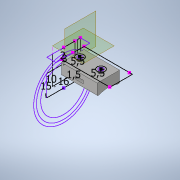
# Autodesk Inventor part: OBS-Displaymountadapter_schmal
Saved by Autodesk Inventor 2021.1 (Build 251245010, 245A)
## iProperties
Created: 2020-11-13
Part Number: OBS-Displaymountadapter_schmal
Material: Generic
Document SubType Name: Modeling
Designer: Administrator
Density: 1 g/cm^3
Appearance: Default
Title: OBS-D-003 v13
Author: Administrator
Autodesk Inventor part; units mm, degrees
ref_plane "YZ Plane" through (0, 0, 0) normal (1, 0, 0) x (0, 1, 0)
ref_plane "XZ Plane" through (0, 0, 0) normal (0, 1, 0) x (-1, 0, 0)
ref_plane "XY Plane" through (0, 0, 0) normal (0, 0, 1) x (1, 0, 0)
ref_plane "Arbeitsebene1" through (-0.5, 0, -8) normal (0, -1, 0) x (1, 0, 0)
sketch "Skizze1" plane through (-0.5, 0, -8) normal (0, -1, 0) x (1, 0, 0)
  line L0 (-6.1, 20) -> (0.5, 20)
  line L1 (0.5, 20) -> (0.5, -4)
  line L2 (0.5, -4) -> (-6.1, -4)
  line L3 (-6.1, -4) -> (-6.1, 20)
  line L4 (0.5, 0) -> (32.9, 0) projected
  line L5 (0.5, 16) -> (34.9, 16) projected
  line L6 (0.5, 0) -> (34.9, 0)
  line L7 (34.9, 0) -> (34.9, 16)
  line L8 (34.9, 16) -> (0.5, 16)
  line L9 (0.5, 16) -> (0.5, 0)
  circle A0 centre (5.5, 8) radius 1.6 projected
  circle A1 centre (5.5, 8) radius 1.6
  circle A2 centre (20.5, 8) radius 1.6 projected
  circle A3 centre (20.5, 8) radius 1.6
  circle A4 centre (5.5, 8) radius 2.75
  circle A5 centre (20.5, 8) radius 2.75
  point P0 (0.5, 8)
  dimension "d0" = 5.5
  dimension "d1" = 5.5
  constraints: 16 end point, 4 centre point, 4 coincident, 4 parallel, 2 horizontal, 2 perpendicular
  measures "d0" diameter of A4
  measures "d1" diameter of A5
extrude "Extrusion1" add sketch "Skizze1" along normal blind 10 contours L0 L1 L2 L3 | L5 L7 L6 L4 L1 | A4 | A5
ref_plane "Arbeitsebene2" through (-6.6, 0, -12) normal (-1, 0, 0) x (0, 0, 1)
sketch "Skizze2" plane through (-6.6, 0, -12) normal (-1, 0, 0) x (0, 0, 1)
  line L0 (0, -10) -> (4, -10) projected
  line L1 (0, -10) -> (24, -10)
  line L2 (24, -10) -> (24, -25)
  line L3 (24, -25) -> (0, -25)
  line L4 (0, -25) -> (0, -10)
  line L5 (0, 0) -> (0, -10) projected
  line L6 (0, 0) -> (4, 0) projected
  line L7 (0, -10) -> (2, -10)
  line L8 (2, -10) -> (2, 0)
  line L9 (2, 0) -> (0, 0)
  line L10 (0, 0) -> (0, -10)
  line L11 (4, 0) -> (4, -10) projected
  line L12 (4, -10) -> (20, -10)
  line L13 (20, -10) -> (20, -20)
  line L14 (20, -20) -> (4, -20)
  line L15 (4, -20) -> (4, -10)
  line L16 (4, -10) -> (5.5, -10)
  line L17 (5.5, -10) -> (5.5, -20)
  line L18 (5.5, -20) -> (4, -20)
  line L19 (4, -20) -> (4, -10)
  circle A0 centre (12, -25) radius 16.3478
  line L20 (12, -8.6522) -> (12, -5.6522)
  line L21 (12, -5.6522) -> (12, -3.6522)
  circle A1 centre (12, -25) radius 19.3478
  circle A2 centre (12, -25) radius 21.3478
  line L22 (4, -20) -> (20, -20)
  line L23 (20, -20) -> (20, 0)
  line L24 (20, 0) -> (4, 0)
  line L25 (4, 0) -> (4, -20)
  point P0 (12, 0)
  point P1 (18.5, -10)
  point P2 (20, -7.3836)
  point P3 (20, -5.2079)
  point P4 (4, -5.2079)
  point P5 (4, -7.3836)
  dimension "d4" = 15
  dimension "d5" = 16
  dimension "d6" = 10
  dimension "d7" = 1.5
  dimension "d14" = 3
  dimension "d15" = 2
  constraints: 44 end point, 10 parallel, 5 horizontal, 5 perpendicular, 2 coincident, 2 midpoint, 2 point on circle, 2 point on line, 1 centre point, 1 vertical, 6 other
  measures "d4" distance of L1.end L2.end
  measures "d5" distance of L13.end L14.end
  measures "d6" distance of L12.end L13.end
  measures "d7" distance of L17.end L18.end
  measures "d14" distance of L20.start L20.end
  measures "d15" distance of L20.end L21.end
extrude "Extrusion2" cut sketch "Skizze2" against normal up to surface (41 mm away) contours A0 L1
sketch "Skizze4" plane through (-0.5, -10, -8) normal (0, -1, 0) x (1, 0, 0)
  circle A0 centre (20.5, 8) radius 1.6 projected
  circle A1 centre (20.5, 8) radius 2.8
  circle A2 centre (5.5, 8) radius 1.6 projected
  circle A3 centre (5.5, 8) radius 2.8
  line L0 (7.1166, 10.8) -> (8.7332, 8)
  line L1 (8.7332, 8) -> (7.1166, 5.2)
  line L2 (7.1166, 5.2) -> (3.8834, 5.2)
  line L3 (3.8834, 5.2) -> (2.2668, 8)
  line L4 (2.2668, 8) -> (3.8834, 10.8)
  line L5 (3.8834, 10.8) -> (7.1166, 10.8)
  line L6 (22.1166, 10.8) -> (23.7332, 8)
  line L7 (23.7332, 8) -> (22.1166, 5.2)
  line L8 (22.1166, 5.2) -> (18.8834, 5.2)
  line L9 (18.8834, 5.2) -> (17.2668, 8)
  line L10 (17.2668, 8) -> (18.8834, 10.8)
  line L11 (18.8834, 10.8) -> (22.1166, 10.8)
  point P0 (0.5, 8)
  point P1 (5.5, 10.8)
  point P2 (20.5, 10.8)
  dimension "d29" = 5.6
  dimension "d30" = 5.6
  constraints: 24 end point, 4 coincident, 2 midpoint, 2 vertical alignment, 1 point on line, 30 other
extrude "Extrusion3" cut sketch "Skizze4" against normal blind 5 contours A0 | A1 | A1 L6 L7 | A1 L11 L6 | L7 L8 A1 | A1 L10 L11 | L8 L9 A1 | A1 L9 L10 | A2 | A3 | A3 L0 L1 | A3 L5 L0 | L1 L2 A3 | A3 L4 L5 | L2 L3 A3 | A3 L3 L4
extrude "Extrusion4" cut sketch "Skizze2" against normal blind 38 contours L11 A2 L21 A1 | A1 L21 A2 L23
extrude "Extrusion5" add sketch "Skizze2" against normal blind 32.5 contours L11 A2 L21 A1 | A1 L21 A2 L23
extrude "Extrusion6" cut sketch "Skizze2" against normal blind 22.05 contours L11 A2 L21 A1 | A1 L21 A2 L23
extrude "Extrusion7" add sketch "Skizze2" against normal blind 16.55 contours L11 A2 L21 A1 | A1 L21 A2 L23
extrude "Extrusion8" cut sketch "Skizze1" along normal blind 16.55 contours A0 | A2
extrude "Extrusion9" cut sketch "Skizze1" along normal blind 2 contours L0 L1 L2 L3 | L5 L7 L6 L4 L1 | A4 | A5
fillet "Rundung1" radius 0.5 9 edges at (-3.3, -10, 12) (0, -10, 10) (17.2, -10, 8) (34.4, -10, 7.25) (34.4, -8.6522, 0) (34.4, -10, -7.25) (17.2, -10, -8) (0, -10, -10) (-3.3, -10, -12)
sketch "Skizze6" plane through (34.4, -2, 8) normal (1, 0, 0) x (0, 0, -1)
  line L0 (-31.6615, 20.7831) -> (48.4189, 20.7831)
  line L1 (48.4189, 20.7831) -> (48.4189, -28.9012)
  line L2 (48.4189, -28.9012) -> (-31.6615, -28.9012)
  line L3 (-31.6615, -28.9012) -> (-31.6615, 20.7831)
  point P0 (8, 2)
  constraints: 8 end point, 2 parallel, 1 horizontal, 1 perpendicular
extrude "Extrusion10" cut sketch "Skizze6" against normal blind 9
sketch "Skizze7" plane through (-6.6, -25, 0) normal (-1, 0, 0) x (0, 0, 1)
  line L0 (-50.9718, 43.6316) -> (27.5939, 43.6316)
  line L1 (27.5939, 43.6316) -> (27.5939, 3.9448)
  line L2 (27.5939, 3.9448) -> (-50.9718, 3.9448)
  line L3 (-50.9718, 3.9448) -> (-50.9718, 43.6316)
  point P0 (0, 25)
  constraints: 8 end point, 2 parallel, 1 horizontal, 1 perpendicular
extrude "Extrusion11" cut sketch "Skizze7" against normal blind 6.6
body "Solid1"
